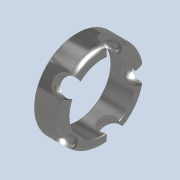
# Autodesk Inventor part: 040205DR-19-H6_cage
Saved by Autodesk Inventor 2021.2 (Build 252289000, 289)
## iProperties
Category: PARTsolutions
Company: TOKBEARING
Part Number: 040205DR-19-H6_cage
Material: 鉄、鋳鉄
Catalog Web Link: www.cadenas.de
Description: DR-H cage-D-Series bearings
Vendor: TOKBEARING
Document SubType Name: Modeling
Designer: partserver
Manufacturer: TOKBEARING
Mass: 8100 g
Surface Area: 3.46761 cm^2
Volume: 0.160981 cm^3
Density: 7.15 g/cm^3
Appearance: 半つや出し
PSOL_IDENT_0: {$CADENAS_DATA\23d-libs\tok_bearing\d_series_bearings\dr_h\dr_h_cage.prj},183 {VTYP=3D},{NB=040205DR
PSOL_IDENT_1: -19-H6_cage},{LINA=040205DR-19-H6_cage},{NN=DR-H cage},{DATE=16.12.2020 00:38:04},{GEOMDATE=03.12.20
PSOL_IDENT_2: 12 14:40:00},{VERSION=},{LINEID=1520},{WBVAR=},{WBNUMERIC=}  {NB=040205DR-19-H6_cage},{LINA=040205DR
PSOL_IDENT_3: -19-H6_cage},{KT=DUMMY},{IDNR=},{CODE=040205},{PN=DR-19-H6},{D=19},{SD=6.0},{W=6},{W1=-},{W1X=0.000}
PSOL_IDENT_4: ,{W2=-},{W2X=0.000},{LOAD=49 (5)},{TYPE=10},{QTY=2.500},{GW=8.1},{BD=3.06},{OP=35.2622},{N=5},{R=5.6
PSOL_IDENT_5: 15},{GP=3.12}
NB: 040205DR-19-H6_cage
NN: DR-H cage
NT: D-Series bearings
NBSYN: $CODE.$PN._cage
LINA: 040205DR-19-H6_cage
CATALOG: TOK, Inc
CODE: 040205
PN: DR-19-H6
D: 19
SD: 6
W: 6
W1: -
W2: -
LOAD: 49 (5)
TYPE: 10
QTY: 2.500
GW: 8.1
SUPPLIER: TOKBEARING
ARTICLENO: 040205DR-19-H6_cage
BOMINFO: 040205DR-19-H6_cage
CREATOR: CADENAS GmbH
Title: 040205DR-19-H6_cage
Author: Cadenas PARTsolutions
Comments: D-Series bearings
Autodesk Inventor part; units mm, degrees
note: some values were not read from the file. Chosen so that the rebuilt part matches the saved one: pattern direction of "Circular Pattern1".
sketch "Sketch_1" plane through (0, 0, 0) normal (0, 0, 1) x (1, 0, 0)
  line L0 (6, 0) -> (2.1, 0)
  arc A0 (2.1, 5.05) -> (2.3, 4.85) centre (2.3, 5.05) ccw
  line L1 (2.3, 4.85) -> (5.8, 4.85)
  arc A1 (5.8, 4.85) -> (6, 5.05) centre (5.8, 5.05) ccw
  line L2 (6, 5.05) -> (6, 6.18)
  arc A2 (6, 6.18) -> (5.8, 6.38) centre (5.8, 6.18) ccw
  line L3 (5.8, 6.38) -> (2.9571, 6.38)
  arc A3 (2.9571, 6.38) -> (2.1, 5.5229) centre (2.9571, 5.5229) ccw
  line L4 (2.1, 5.5229) -> (2.1, 5.05)
  constraints: 10 end point, 8 point on circle, 4 centre point
revolve "Revolution1" add sketch "Sketch_1" angle 360 about axis through (6, 0, 0) along (1, 0, 0)
sketch "Sketch_2" plane through (3, 0, 0) normal (1, 0, 0) x (0, 0, -1)
  line L0 (0, 7.145) -> (0, 4.085)
  arc A0 (0, 7.145) -> (0, 4.085) centre (0, 5.615) ccw
  line L1 (0, 7.145) -> (0, 4.085)
  constraints: 4 end point, 2 point on circle, 1 centre point
revolve "Revolution2" cut sketch "Sketch_2" angle 360 about axis through (3, 7.145, 0) along (0, 1, 0)
pattern_circular "Circular Pattern1" count 5 over 360 about axis through (3, 0, 0) along (1, 0, 0) of "Revolution2"
ref_plane "Cage_OR_XY" through (0, 0, 0) normal (1, 0, 0) x (0, 0, -1)
ref_plane "Cage_OR_YZ" through (0, 0, 0) normal (0, 0, -1) x (0, 1, 0)
ref_plane "Cage_OR_ZX" through (0, 0, 0) normal (0, 1, 0) x (1, 0, 0)
body "Solid1"
